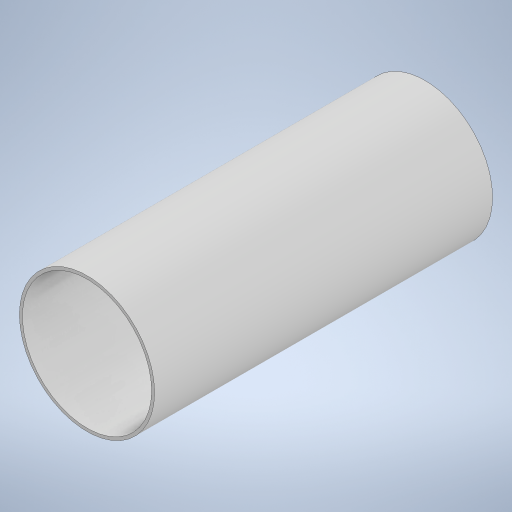
# Autodesk Inventor part: Tambor liso (drum)
Saved by Autodesk Inventor 2024.3 (Build 283343000, 343)
## iProperties
Created: 2025-07-02
Part Number: Tambor liso (drum)
Material: Genérico
Document SubType Name: Modeling
Designer: Daniel Rodriguez
Density: 1 g/cm^3
Appearance: Valor por defecto
Author: Daniel Rodriguez
Autodesk Inventor part; units mm, degrees
ref_plane "YZ Plane" through (0, 0, 0) normal (1, 0, 0) x (0, 1, 0)
ref_plane "XZ Plane" through (0, 0, 0) normal (0, 1, 0) x (-1, 0, 0)
ref_plane "XY Plane" through (0, 0, 0) normal (0, 0, 1) x (1, 0, 0)
sketch "Boceto1" plane through (0, 0, 0) normal (0, 0, 1) x (1, 0, 0)
  circle A0 centre (0, 0) radius 325
  circle A1 centre (0, 0) radius 340
  dimension "d0" = 680
  dimension "d1" = 650
  constraints: 2 centre point, 2 coincident
  measures "d0" diameter of A1
  measures "d1" diameter of A0
extrude "Extrusión1" add sketch "Boceto1" along normal mid plane 1700
